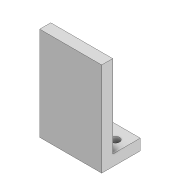
# Autodesk Inventor part: BatteryMount
Saved by Autodesk Inventor 2022 (Build 260153000, 153)
## iProperties
Created: 2022-10-26
Part Number: BatteryMount
Material: Generic
Document SubType Name: Modeling
Designer: MVeszpremi
Density: 1 g/cm^3
Appearance: Default
Author: MVeszpremi
Autodesk Inventor part; units mm, degrees
ref_plane "YZ Plane" through (0, 0, 0) normal (1, 0, 0) x (0, 1, 0)
ref_plane "XZ Plane" through (0, 0, 0) normal (0, 1, 0) x (-1, 0, 0)
ref_plane "XY Plane" through (0, 0, 0) normal (0, 0, 1) x (1, 0, 0)
sketch "Sketch1" plane through (0, 0, 0) normal (0, 1, 0) x (-1, 0, 0)
  line L0 (0, 0) -> (22.5, 0)
  line L1 (22.5, 0) -> (22.5, -10)
  line L2 (22.5, -10) -> (0, -10)
  line L3 (0, -10) -> (0, 0)
  circle A0 centre (19, -5) radius 1.5
  circle A1 centre (4, -5) radius 1.5
  dimension "d0" = 3
  dimension "d1" = 3
  dimension "d2" = 22.5
  dimension "d3" = 15
  dimension "d4" = 5
  dimension "d5" = 10
  dimension "d6" = 3.5
  constraints: 8 end point, 2 centre point, 2 parallel, 1 horizontal, 1 horizontal alignment, 1 perpendicular
  measures "d0" diameter of A0
  measures "d1" diameter of A1
  measures "d2" distance of L1.end L2.end
  measures "d3" distance of A1.centre A0.centre
  measures "d4" distance from line of L0 A0.centre
  measures "d5" distance of L0.end L1.end
  measures "d6" distance from line of L1 A0.centre
extrude "Extrusion1" add sketch "Sketch1" along normal blind 4
sketch "Sketch2" plane through (0, 4, 0) normal (0, 1, 0) x (1, 0, 0)
  line L0 (-22.5, 0) -> (0, 0) projected
  line L1 (0, 0) -> (-22.5, 0)
  line L2 (-22.5, 0) -> (-22.5, -4)
  line L3 (-22.5, -4) -> (0, -4)
  line L4 (0, -4) -> (0, 0)
  dimension "d9" = 4
  constraints: 8 end point, 2 parallel, 1 horizontal, 1 perpendicular
  measures "d9" distance of L3.end L0.end
extrude "Extrusion2" add sketch "Sketch2" along normal blind 30 and the other way blind 4
body "Solid1"
